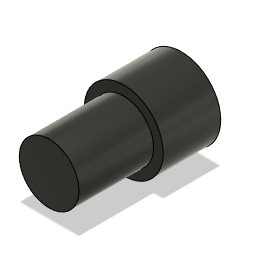
EGR314_Team_305_Blinds_Demo_ (Autodesk Fusion 360 archive; units mm, degrees)
design "Motor"
Autodesk Fusion 360 part; units mm, degrees
sketch "Sketch1" plane through (0, 0, 0) normal (0, 0, 1) x (1, 0, 0)
  circle A0 centre (0, 0) radius 18.5
  dimension "d1" = 37
  constraint coincident A0.centre origin
  measures "d1" diameter of A0
extrude "Extrude1" add sketch "Sketch1" along normal blind 27 makes body 1
sketch "Sketch2" plane through (0, 0, 27) normal (0, 0, 1) x (1, 0, 0)
  circle A0 centre (0, 0) radius 18.5
  circle A1 centre (0, 0) radius 14
  dimension "d4" = 28
  constraint coincident A0.centre A1.centre
  measures "d4" diameter of A1
extrude "Extrude2" add sketch "Sketch2" along normal blind 35 contours A1 bodies 1
sketch "Sketch3" plane through (0, 0, 0) normal (0, 0, -1) x (-1, 0, 0)
  circle A0 centre (0, 0) radius 18.5
  circle A1 centre (0, 0) radius 6
  dimension "d7" = 12
  constraint coincident A0.centre A1.centre
  measures "d7" diameter of A1
extrude "Extrude3" add sketch "Sketch3" along normal blind 3 contours A1 bodies 1
fillet "Fillet1" radius 0.5 1 edges at (5.594, -2.1697, -3) on bodies 1
sketch "Sketch4" plane through (0, 0, -3) normal (0, 0, -1) x (-1, 0, 0)
  circle A0 centre (0, 0) radius 5.5
  circle A1 centre (0, 0) radius 3
  dimension "d12" = 6
  constraint concentric A0 A1
  measures "d12" diameter of A1
extrude "Extrude4" add sketch "Sketch4" along normal blind 9 contours A1 bodies 1
ref_plane "WorkPlane1" through (0, 0, 0) normal (0, 0, -1) x (-1, 0, 0)
split "Split1" by plane through (0, 0, 0) normal (0, 0, -1) bodies 1 makes body 2 at (-2.9963, -0.1495, -9)
sketch "Sketch5" plane through (0, 0, 0) normal (0, 0, -1) x (1, 0, 0)
  circle A0 centre (0, 0) radius 18.5
  line L0 (0, 18.5) -> (0, 13.5)
  dimension "d16" = 37
  dimension "d17" = 5
  constraint coincident A0.centre origin
  constraint coincident A0 L0.start
  measures "d16" diameter of A0
  measures "d17" distance of L0.start L0.end
move_body "Move1" bodies 2 to x (1, 0, 0) y (0, 1, 0) z (0, 0, 1) at (0, -13.5, 0)
move_body "Move2" bodies 2 to x (1, 0, 0) y (0, 1, 0) z (0, 0, 1) at (0, 6, 0)
combine "Combine1" operation add target body 1 tool bodies 2
